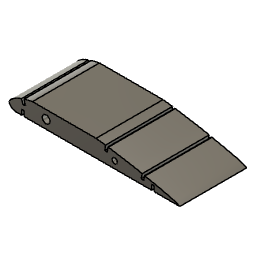
Wing section for 3d printing v1 (Autodesk Fusion 360 design; units mm, degrees)
Autodesk Fusion 360 part; units mm, degrees
sketch "Sketch1" plane through (0, 0, 0) normal (0, 0, 1) x (1, 0, 0) in component "Airfoil structure"
  spline S0 degree 5 poles (108.4359, 17.4637) (108.6467, 17.433) (108.9931, 17.3831) (109.2865, 17.3426) (109.4924, 17.3142) (110.5153, 17.1479) (112.7968, 16.7722) (116.3555, 16.1857) (120.8901, 15.4386) (125.9027, 14.6124) (130.8234, 13.7994) (135.1309, 13.0827) (138.47, 12.5166) (140.7881, 12.1042) (142.4392, 11.78) (143.9897, 11.4433) (145.6466, 11.0766) (147.3521, 10.7068) (148.7253, 10.4127) (149.471, 10.2539) knots 0 0 0 0 0 0 0.066667 0.133333 0.2 0.266667 0.333333 0.4 0.466667 0.533333 0.6 0.666667 0.733333 0.8 0.866667 0.933333 1 1 1 1 1 1
  line L0 (104.3135, 18.0638) -> (112.5583, 16.8636)
  line L1 (145.493, 11.1014) -> (153.4489, 9.4063)
  spline S1 degree 5 poles (152.8506, 9.5306) (153.6754, 9.3537) (155.1958, 9.0287) (157.0885, 8.6275) (158.936, 8.2427) (160.6637, 7.8881) (162.4454, 7.5151) (164.8303, 6.998) (168.0437, 6.2836) (171.9513, 5.3996) (176.2204, 4.4167) (180.4193, 3.4264) (184.1364, 2.5129) (187.0894, 1.7283) (189.2467, 1.0645) (190.9412, 0.4268) (192.3181, -0.1665) (193.5665, -0.7111) (194.5238, -1.126) (195.0337, -1.3464) knots 0 0 0 0 0 0 0.066667 0.133333 0.2 0.266667 0.333333 0.4 0.466667 0.533333 0.6 0.666667 0.733333 0.8 0.866667 0.933333 1 1 1 1 1 1
  line L2 (148.4907, 10.4656) -> (157.2105, 8.5955)
  line L3 (191.9852, -0.0289) -> (198.0822, -2.6639)
  circle A0 centre (33.1388, 9.1296) radius 4.765
  circle A1 centre (116.1615, 7.0362) radius 3.175
  spline S2 degree 5 poles (-3.081, -1.3464) (-3.6016, -1.2536) (-4.5414, -1.0763) (-5.6463, -0.8353) (-6.5938, -0.5669) (-7.329, -0.2953) (-8.0513, 0.0089) (-9.0194, 0.5707) (-10.0683, 1.7874) (-10.9642, 3.2518) (-11.5103, 4.4866) (-11.5777, 5.0951) (-11.407, 5.643) (-11.0112, 6.6067) (-10.1307, 7.993) (-8.6022, 9.6431) (-6.4035, 11.272) (-4.1965, 12.5715) (-2.7349, 13.4061) (-1.8316, 13.8946) (-1.0216, 14.2664) (0.0955, 14.6934) (1.459, 15.1916) (2.6392, 15.6173) (3.2971, 15.8534) knots 0 0 0 0 0 0 0.05 0.1 0.15 0.2 0.25 0.3 0.35 0.4 0.45 0.5 0.55 0.6 0.65 0.7 0.75 0.8 0.85 0.9 0.95 1 1 1 1 1 1
  line L4 (0.5703, -1.9971) -> (-6.7323, -0.6957)
  line L5 (-0.0118, 14.6656) -> (6.606, 17.0412)
  line L6 (-8.4792, 9.8153) -> (-3.9569, 12.8132)
  line L7 (-11.5034, 4.2257) -> (-11.5345, 5.6935)
  line L8 (-7.2174, -0.5359) -> (-9.7443, 1.1286)
  line L9 (16.5688, 19.3646) -> (93.5688, 19.3646)
  spline S3 degree 5 poles (93.5688, 19.3646) (93.8188, 19.3387) (94.2829, 19.2905) (94.8714, 19.229) (95.4658, 19.1659) (96.0263, 19.1049) (96.567, 19.0445) (97.2368, 18.9678) (98.1315, 18.8622) (99.313, 18.7173) (100.8214, 18.5245) (102.3118, 18.3263) (103.5973, 18.1504) (104.53, 18.0207) (105.0153, 17.9528) knots 0 0 0 0 0 0 0.1 0.2 0.3 0.4 0.5 0.6 0.7 0.8 0.9 1 1 1 1 1 1
  line L10 (92.266, 19.4996) -> (94.8715, 19.2297)
  line L11 (103.6448, 18.1447) -> (106.3858, 17.761)
  spline S4 degree 5 poles (6.5765, 16.943) (6.9079, 17.0449) (7.5374, 17.2364) (8.3817, 17.4868) (9.3156, 17.7508) (10.2084, 17.9865) (10.8922, 18.156) (11.4504, 18.29) (11.9864, 18.4184) (12.6265, 18.5675) (13.504, 18.76) (14.4962, 18.9637) (15.447, 19.1503) (16.1786, 19.2906) (16.5688, 19.3646) knots 0 0 0 0 0 0 0.1 0.2 0.3 0.4 0.5 0.6 0.7 0.8 0.9 1 1 1 1 1 1
  line L12 (5.4107, 16.5846) -> (7.7424, 17.3015)
  line L13 (15.2328, 19.111) -> (17.9048, 19.6183)
  line L14 (152.4045, 9.626) -> (152.8506, 9.5306)
  line L15 (107.9851, 17.5282) -> (108.4359, 17.4637)
  line L16 (6.1441, 16.7993) -> (6.5765, 16.943)
  line L17 (128.8588, -1.3464) -> (132.3138, -1.3464)
  line L18 (132.3138, -1.3464) -> (160.8934, -1.3464)
  line L19 (163.8934, -1.3464) -> (195.0337, -1.3464)
  line L20 (-3.081, -1.3464) -> (3.4513, -1.3464)
  line L21 (6.4513, -1.3464) -> (128.8588, -1.3464)
  line L22 (107.9851, 17.5282) -> (107.1357, 11.5886)
  line L23 (107.1357, 11.5886) -> (104.166, 12.0132)
  line L24 (104.166, 12.0132) -> (105.0153, 17.9528)
  line L25 (152.4045, 9.626) -> (151.1489, 3.7589)
  line L26 (151.1489, 3.7589) -> (148.2153, 4.3867)
  line L27 (148.2153, 4.3867) -> (149.471, 10.2539)
  line L28 (160.8934, -1.3464) -> (160.8934, 4.6536)
  line L29 (160.8934, 4.6536) -> (163.8934, 4.6536)
  line L30 (163.8934, 4.6536) -> (163.8934, -1.3464)
  line L31 (3.4513, -1.3464) -> (3.4513, 4.6536)
  line L32 (6.4513, -1.3464) -> (6.4513, 4.6536)
  line L33 (3.4513, 4.6536) -> (6.4513, 4.6536)
  line L34 (6.1441, 16.7993) -> (8.0359, 11.1054)
  line L35 (8.0359, 11.1054) -> (5.1889, 10.1595)
  line L36 (3.2971, 15.8534) -> (5.1889, 10.1595)
  point P0 (-8.4808, 0.2964)
  point P1 (-11.5189, 4.9596)
  point P2 (-6.2181, 11.3142)
  point P3 (11.4183, 18.2822)
  point P4 (96.5722, 19.0435)
  point P5 (109.7229, 17.2753)
  point P6 (137.8507, 12.6179)
  point P7 (163.7248, 7.2358)
  point P8 (186.791, 1.7868)
  dimension "d38" = 77
  dimension "d53" = 9.53
  dimension "d54" = 6.35
  dimension "d56" = 6
  dimension "d57" = 3
  dimension "d58" = 6
  dimension "d59" = 3
  dimension "d60" = 6
  dimension "d61" = 3
  dimension "d62" = 6
  dimension "d63" = 6
  constraint midpoint S0.start L0
  constraint midpoint S0.end L1
  constraint midpoint S1.start L2
  constraint midpoint S1.end L3
  constraint midpoint S2.start L4
  constraint midpoint S2.end L5
  constraint midpoint P2 L6
  constraint midpoint P1 L7
  constraint midpoint P0 L8
  constraint horizontal L9
  constraint midpoint L9.end L10
  constraint midpoint S3.end L11
  constraint midpoint S4.start L12
  constraint midpoint L9.start L13
  constraint parallel L18 L20
  constraint collinear L18 L20
  constraint horizontal L20
  constraint parallel L17 L18
  constraint collinear L18 L19
  constraint coincident L21.start L20
  constraint collinear L20 L21
  constraint perpendicular L15 L22
  constraint perpendicular L22 L23
  constraint perpendicular L23 L24
  constraint perpendicular L14 L25
  constraint perpendicular L25 L26
  constraint perpendicular L26 L27
  constraint perpendicular L18 L28
  constraint perpendicular L28 L29
  constraint perpendicular L19 L30
  constraint perpendicular L20 L31
  constraint perpendicular L21 L32
  constraint perpendicular L32 L33
  constraint perpendicular L16 L34
  constraint perpendicular L34 L35
  constraint perpendicular L35 L36
  measures "d38" distance of L9.start L9.end
  measures "d53" diameter of A0
  measures "d54" diameter of A1
  measures "d56" distance of L15.start L22.end
  measures "d57" distance of L22.end L23.end
  measures "d58" distance of L14.start L25.end
  measures "d59" distance of L25.end L26.end
  measures "d60" distance of L18.end L28.end
  measures "d61" distance of L28.end L29.end
  measures "d62" distance of L20.end L31.end
  measures "d63" distance of L21.start L32.end
extrude "Extrude2" add sketch "Sketch1" along normal blind 81.1111 contours S0 L0 S1 L2 L3 S2 L9 S3 L10 L11 S4 L14 L15 L16 L17 L18 L19 L20 L21 L22 L23 L24 L25 L26 L27 L28 L29 L30 L31 L32 L33 L34 L35 L36
sketch "Sketch3" plane through (0, 0, 0) normal (0, 0, 1) x (1, 0, 0)
component "Airfoil structure" placed x (1, 0, 0) y (0, 1, 0) z (0, 0, 1) at (0, 0, 0)
